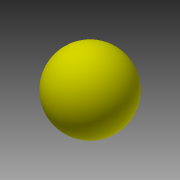
# Autodesk Inventor part: 61814-2RS1_PART3
Saved by Autodesk Inventor 2014 SP2 (Build 180246200, 246)
## iProperties
Created: 2019-11-07
Part Number: 61814-2RS1_PART3
Material: Generic
Catalog Web Link: www.cadenas.de
Description: -Deep groove ball bearings
Vendor: SKF
Document SubType Name: Modeling
Designer: psadmin
Manufacturer: SKF
Mass: 0.0898019 g
Surface Area: 0.969783 cm^2
Volume: 0.0898019 cm^3
Density: 1 g/cm^3
Appearance: PSOLRGB-192-192-192
Category: PARTsolutions
Company: SKF
Title: 61814-2RS1_PART3
Author: Cadenas PARTsolutions
Comments: Deep groove ball bearings
PSOL_IDENT_0: {$CADENAS_DATA\23d-libs\skf\bearings_units_and_housings\ball_bearings\deep_groove_ball_bearings\bb1_
PSOL_IDENT_1: 001_101.prj},198 {VTYP=3D},{NB=61814-2RS1_PART3},{LINA=61814-2RS1_PART3},{NN=BB1_001_101_PART3},{NOP
PSOL_IDENT_2: RJ=TRUE},{DATE=07.11.2019 10:38:24},{GEOMDATE=11.06.2019 11:24:58},{VERSION=},{LINEID=8240},{WBVAR=}
PSOL_IDENT_3: ,{WBNUMERIC=}  {NB=61814-2RS1_PART3},{LINA=61814-2RS1_PART3},{KT=DUMMY},{PRODUCTID=1010271814},{DESI
PSOL_IDENT_4: GNATION=61814-2RS1},{DD=70.00},{D=90.000},{B=10.000},{C=0.000},{DD1=76.40},{DD2=0.0},{D1=0.00},{D2=8
PSOL_IDENT_5: 5.50},{D3=0.00},{D4=0.000},{HH=MIN},{BB=0.000},{FF=0.00},{R0MAX=MIN},{R0=MIN},{R12=0.60},{PITCH=80.0
PSOL_IDENT_6: 0},{DW=5.556},{DDAMIN=73.200},{DDAMAX=76.500},{DDBMIN=MIN},{DDBMAX=MIN},{DBMIN=MIN},{DAMAX=86.800},{
PSOL_IDENT_7: BBAMIN=MIN},{CAMAX=MIN},{RAMAX=0.600},{LOAD1=12.400},{LOAD2=13.200},{LOAD3=0.560},{SPEED1=MIN},{SPEE
PSOL_IDENT_8: D2=4300},{KR=0.015},{F0=17.200},{Z=24},{II=1},{MASS=0.140},{BEARING=61814-2RS1},{RING=},{HELP=3.139}
PSOL_IDENT_9: ,{HELP2=2.250},{DD1ALG=38.200},{YALG=38.200},{PITCH1=80.000},{DW1=5.556},{YALG1=41.861},{HALG1=3.139
PSOL_IDENT_10: },{SH=38.200},{CU=0.889},{DESIGN=dgbb2rs},{HALG=3.2},{B1=0},{ALGO=1.000}
NT: Deep groove ball bearings
NB: 61814-2RS1_PART3
NBSYN: $DESIGNATION._PART3
LINA: 61814-2RS1_PART3
SUPPLIER: SKF
ARTICLENO: 61814-2RS1_PART3
BOMINFO: 61814-2RS1_PART3
CREATOR: CADENAS GmbH
Autodesk Inventor part; units mm, degrees
ref_plane "YZ Plane" through (0, 0, 0) normal (1, 0, 0) x (0, 1, 0)
ref_plane "XZ Plane" through (0, 0, 0) normal (0, 1, 0) x (-1, 0, 0)
ref_plane "XY Plane" through (0, 0, 0) normal (0, 0, 1) x (1, 0, 0)
sketch "Sketch_6" plane through (0, 0, 0) normal (0, 0, 1) x (1, 0, 0)
  line L0 (7.778, 40) -> (2.222, 40)
  arc A0 (7.778, 40) -> (2.222, 40) centre (5, 40) ccw
  line L1 (7.778, 40) -> (2.222, 40)
  dimension "d0" = 360
  constraints: 4 end point, 2 point on circle, 1 centre point
revolve "Revolution1" add sketch "Sketch_6" angle 360 about axis through (7.778, 40, 0) along (1, 0, 0)
body "Solid1"
